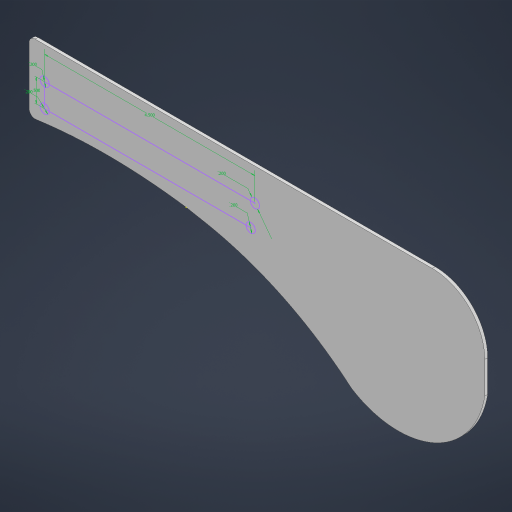
# Autodesk Inventor part: meers goofy intake sled
Saved by Autodesk Inventor 2023.4 (Build 274418000, 418)
## iProperties
Created: 2023-12-16
Part Number: meers goofy intake sled
Material: Generic
Document SubType Name: Modeling
Designer: Meer
Density: 1 g/cm^3
Appearance: Default
Author: Meer
Autodesk Inventor part; units mm, degrees
ref_plane "YZ Plane" through (0, 0, 0) normal (1, 0, 0) x (0, 1, 0)
ref_plane "XZ Plane" through (0, 0, 0) normal (0, 1, 0) x (-1, 0, 0)
ref_plane "XY Plane" through (0, 0, 0) normal (0, 0, 1) x (1, 0, 0)
sketch "Sketch1" plane through (0, 0, 0) normal (0, 0, 1) x (1, 0, 0)
  line L0 (-85.3538, 38.1) -> (162.2962, 38.1)
  line L1 (162.2962, 38.1) -> (162.2962, 12.7)
  line L2 (162.2962, 12.7) -> (-85.3538, 12.7)
  line L3 (-85.3538, 12.7) -> (-85.3538, 38.1)
  line L4 (162.2962, 38.1) -> (115.3062, 38.1)
  line L5 (115.3062, 38.1) -> (115.3062, 0)
  line L6 (115.3062, 0) -> (162.2962, 0)
  line L7 (162.2962, 0) -> (162.2962, 38.1)
  circle A0 centre (-22.5792, -171.9682) radius 173.1686
  line L8 (-85.3538, 12.7) -> (-85.3538, 0)
  line L9 (0, 0) -> (-44.3742, 6.35) construction
  line L10 (-44.3742, 6.35) -> (-85.3538, 0) construction
  spline S0 degree 2 poles (0, 0) (-44.3742, 6.35) (-85.3538, 0) knots 1 1 1 2 2 2
  line L11 (81.5863, -33.6319) -> (69.4058, 12.7)
  line L12 (0, 0) -> (0, 12.7)
  line L13 (0, 0) -> (67.6812, 0)
  line L14 (0, 0) -> (67.6812, 0)
  line L15 (81.5863, -33.6319) -> (29.3756, 0)
  line L16 (0, 0) -> (29.3756, 0)
  line L17 (27.7818, -6.2843) -> (29.3756, 0)
  line L18 (27.7744, -6.2821) -> (21.0977, 0)
  line L19 (7.9763, 0) -> (27.7808, -6.2881)
  line L20 (7.9763, 0) -> (7.5205, -1.4355)
  line L21 (0, 0) -> (7.5205, -1.4355) construction
  spline S1 degree 1 poles (0, 0) (7.5205, -1.4355) knots 1 1 2 2
  line L22 (81.5863, -33.6319) -> (101.3506, -50.0871) construction
  line L23 (101.3506, -50.0871) -> (95.7634, -43.4306) construction
  spline S2 degree 2 poles (81.5863, -33.6319) (101.3506, -50.0871) (95.7634, -43.4306) knots 1 1 1 2 2 2
  line L24 (162.2962, 0) -> (162.2962, -7.7512)
  arc A1 (88.9377, -39.659) -> (162.2962, -7.7512) centre (115.3062, 0) ccw
  arc A2 (162.2962, 7.7512) -> (81.5863, -33.6319) centre (115.3062, 0) ccw
  point P0 (60.3061, -19.9241)
  point P1 (162.2962, 12.7)
  point P2 (115.3062, 12.7)
  point P3 (162.2962, 12.7)
  point P4 (27.497, -6.198)
  point P5 (29.3756, 0)
  point P6 (89.8079, -40.2241)
  dimension "d0" = 247.65
  dimension "d1" = 25.4
  dimension "d4" = 38.1
  dimension "d5" = 46.99
  constraints: 40 end point, 11 point on circle, 9 point on line, 5 equal length, 5 perpendicular, 3 centre point, 2 coincident, 2 horizontal, 1 vertical, 10 other
  measures "d0" distance of L0.start L0.end
  measures "d1" distance of L2.end L0.start
  measures "d4" distance of L4.end L5.end
  measures "d5" distance of L5.end L6.end
extrude "Extrusion2" add sketch "Sketch1" along normal blind 1.5875 contours L0 A2 L2 L3 | L0 L5 L2 A2 | L2 L12 S0 L8 | L0 A2 L2 L5 | L0 L1 L2 A2 | A2 L13 L12 L2 | L2 L5 L6 L24 A1 A0 L11 | L11 A2 | L2 A2 L7 L6 L5 | L2 L7 A2 | A0 L15 L13 A2 | L13 L20 S1 | A0 L17 L15 | L17 A0 L18 L13 | L13 L18 A0 L19 | L19 A0 L20
fillet "Fillet1" radius 28.575 1 edges at (162.2962, 38.1, 0.7937)
fillet "Fillet2" radius 3.175 1 edges at (-85.3538, 38.1, 0.7937)
fillet "Fillet3" radius 3.175 1 edges at (-85.3538, 0, 0.7937)
sketch "Sketch2" plane through (0, 0, 1.5875) normal (0, 0, 1) x (1, 0, 0)
  circle A0 centre (-77.0322, 20.6187) radius 2.54
  line L0 (-77.0322, 20.6187) -> (-77.0322, 7.9187)
  circle A1 centre (-77.0322, 7.9187) radius 2.54
  line L1 (-77.0322, 20.6187) -> (37.2678, 20.6187)
  circle A2 centre (37.2678, 20.6187) radius 2.54
  line L2 (-77.0322, 7.9187) -> (34.9936, 7.9187)
  circle A3 centre (34.9936, 7.9187) radius 2.54
  point P0 (0, 0)
  dimension "d15" = 5.08
  dimension "d16" = 12.7
  dimension "d17" = 5.08
  dimension "d18" = 114.3
  dimension "d19" = 5.08
  dimension "d20" = 5.08
  constraints: 6 end point, 4 centre point, 3 coincident, 2 horizontal, 1 vertical
  measures "d15" diameter of A0
  measures "d16" distance of L0.start L0.end
  measures "d17" diameter of A1
  measures "d18" distance of L0.start L1.end
  measures "d19" diameter of A2
  measures "d20" diameter of A3
body "Solid2"
